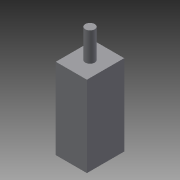
# Autodesk Inventor part: motor
Saved by Autodesk Inventor 2015 (Build 190159000, 159)
## iProperties
Created: 2014-10-24
Part Number: motor
Material: Generic
Document SubType Name: Modeling
Designer: Colin
Density: 1 g/cm^3
Appearance: Default
Author: Colin
Autodesk Inventor part; units mm, degrees
ref_plane "YZ Plane" through (0, 0, 0) normal (1, 0, 0) x (0, 1, 0)
ref_plane "XZ Plane" through (0, 0, 0) normal (0, 1, 0) x (-1, 0, 0)
ref_plane "XY Plane" through (0, 0, 0) normal (0, 0, 1) x (1, 0, 0)
sketch "Sketch2" plane through (0, 0, 0) normal (0, 1, 0) x (-1, 0, 0)
  line L0 (0, 0) -> (-10, 0)
  line L1 (-10, 0) -> (-10, -12)
  line L2 (-10, -12) -> (0, -12)
  line L3 (0, -12) -> (0, 0)
  dimension "d3" = 12
  dimension "d4" = 10
  constraints: 8 end point, 2 parallel, 1 horizontal, 1 perpendicular
  measures "d3" distance of L0.end L1.end
  measures "d4" distance of L1.end L2.end
extrude "Extrusion1" add sketch "Sketch2" along normal blind 26
sketch "Sketch3" plane through (0, 26, 0) normal (0, 1, 0) x (1, 0, 0)
  line L0 (0, 12) -> (0, 0) projected
  line L1 (0, 6) -> (10, 6) construction
  line L2 (10, 0) -> (10, 12) projected
  line L3 (0, 0) -> (10, 0) projected
  line L4 (5, 0) -> (5, 12) construction
  line L5 (10, 12) -> (0, 12) projected
  circle A0 centre (5, 6) radius 1.5
  dimension "d9" = 3
  constraints: 5 midpoint, 4 end point, 1 centre point
  measures "d9" diameter of A0
extrude "Extrusion2" add sketch "Sketch3" along normal blind 9.27 contours A0
body "Solid1"
